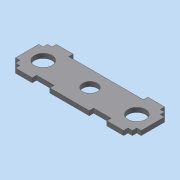
# Autodesk Inventor part: Bearing-Outer
Saved by Autodesk Inventor 2016 SP1 (Build 200210100, 210)
## iProperties
Created: 2016-03-01
Part Number: Bearing-Outer
Material: Generic
Document SubType Name: Modeling
Designer: Mohamed A.
Density: 1 g/cm^3
Appearance: Default
Author: Mohamed A.
Autodesk Inventor part; units mm, degrees
ref_plane "YZ Plane" through (0, 0, 0) normal (1, 0, 0) x (0, 1, 0)
ref_plane "XZ Plane" through (0, 0, 0) normal (0, 1, 0) x (-1, 0, 0)
ref_plane "XY Plane" through (0, 0, 0) normal (0, 0, 1) x (1, 0, 0)
sketch "Sketch2" plane through (0, 0, 0) normal (0, 0, 1) x (1, 0, 0)
  circle A0 centre (-32, 0) radius 7.5 construction
  circle A1 centre (32, 0) radius 7.5 construction
  circle A2 centre (0, 0) radius 5 projected
  line L0 (-13.5, 14) -> (13.5, 14) projected
  line L1 (13.5, 14) -> (13.5, 11) projected
  line L2 (13.5, 11) -> (25.5, 11) projected
  line L3 (25.5, 11) -> (25.5, 14) projected
  line L4 (25.5, 14) -> (37, 14) projected
  line L5 (37, 14) -> (37, 11) projected
  line L6 (37, 11) -> (40, 11) projected
  line L7 (40, 11) -> (40, 8) projected
  line L8 (40, 8) -> (43, 8) projected
  line L9 (43, 8) -> (43, -8) projected
  line L10 (43, -8) -> (40, -8) projected
  line L11 (40, -8) -> (40, -11) projected
  line L12 (40, -11) -> (37, -11) projected
  line L13 (37, -11) -> (37, -14) projected
  line L14 (37, -14) -> (25.5, -14) projected
  line L15 (25.5, -14) -> (25.5, -11) projected
  line L16 (25.5, -11) -> (13.5, -11) projected
  line L17 (13.5, -11) -> (13.5, -14) projected
  line L18 (13.5, -14) -> (-13.5, -14) projected
  line L19 (-13.5, -14) -> (-13.5, -11) projected
  line L20 (-13.5, -11) -> (-25.5, -11) projected
  line L21 (-25.5, -11) -> (-25.5, -14) projected
  line L22 (-25.5, -14) -> (-37, -14) projected
  line L23 (-37, -14) -> (-37, -11) projected
  line L24 (-37, -11) -> (-40, -11) projected
  line L25 (-40, -11) -> (-40, -8) projected
  line L26 (-40, -8) -> (-43, -8) projected
  line L27 (-43, -8) -> (-43, 8) projected
  line L28 (-43, 8) -> (-40, 8) projected
  line L29 (-40, 8) -> (-40, 11) projected
  line L30 (-40, 11) -> (-37, 11) projected
  line L31 (-37, 11) -> (-37, 14) projected
  line L32 (-37, 14) -> (-25.5, 14) projected
  line L33 (-25.5, 14) -> (-25.5, 11) projected
  line L34 (-25.5, 11) -> (-13.5, 11) projected
  line L35 (-13.5, 11) -> (-13.5, 14) projected
  circle A3 centre (-32, 0) radius 6
  circle A4 centre (32, 0) radius 6
  line L36 (25.5, 11) -> (-25.5, 11)
  line L37 (-25.5, 14) -> (-25.5, 11)
  line L38 (-25.5, 14) -> (-37, 14)
  line L39 (-37, 11) -> (-37, 14)
  line L40 (-37, 11) -> (-40, 11)
  line L41 (-40, 8) -> (-40, 11)
  line L42 (-40.3391, 8) -> (-43, 8)
  line L43 (-43, -8) -> (-43, 8)
  line L44 (-43, -8) -> (-40, -8)
  line L45 (-40, -11) -> (-40, -8)
  line L46 (-40, -11) -> (-37, -11)
  line L47 (-37, -11) -> (-37, -14)
  line L48 (-37, -14) -> (-25.5, -14)
  line L49 (-25.5, -11) -> (-25.5, -14)
  line L50 (-25.5, -11) -> (-13.5, -11)
  line L51 (-13.5, -11) -> (-13.5, -14)
  line L52 (13.5, -14) -> (-13.5, -14)
  line L53 (13.5, -11) -> (13.5, -14)
  line L54 (13.5, -11) -> (25.5, -11)
  line L55 (25.5, -11) -> (25.5, -14)
  line L56 (25.5, -14) -> (37, -14)
  line L57 (37, -11) -> (37, -14)
  line L58 (37, -11) -> (40, -11)
  line L59 (40, -11) -> (40, -8)
  line L60 (40, -8) -> (43, -8)
  line L61 (43, -8) -> (43, 8)
  line L62 (43, 8) -> (40, 8)
  line L63 (40, 8) -> (40, 11)
  line L64 (37, 11) -> (40, 11)
  line L65 (37, 11) -> (37, 14)
  line L66 (37, 14) -> (25.5, 14)
  line L67 (25.5, 14) -> (25.5, 11)
  dimension "d11" = 12
  dimension "d12" = 12
  constraints: 64 end point, 27 collinear, 5 perpendicular, 2 centre point, 2 coincident, 1 point on line
  measures "d11" diameter of A3
  measures "d12" diameter of A4
extrude "Extrusion1" add sketch "Sketch2" along normal blind 3 contours L36 L2 L3 L4 L5 L6 L7 L8 L9 L10 L11 L12 L13 L14 L15 L16 L17 L18 L19 L20 L21 L22 L23 L24 L25 L26 L27 L28 L29 L30 L31 L32 L33 L34
body "Solid1"
